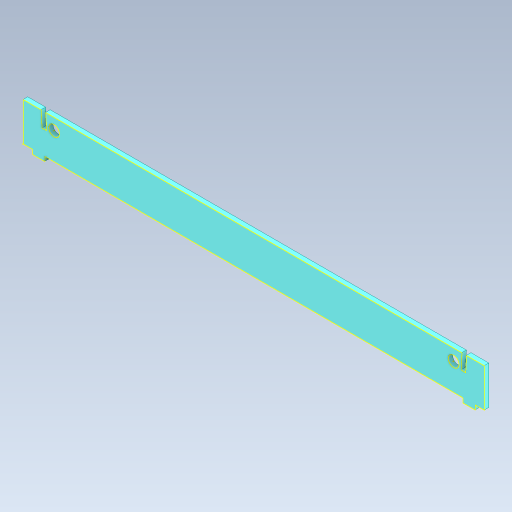
# Autodesk Inventor part: 零件1
Saved by Autodesk Inventor 2023 (Build 270158000, 158)
## iProperties
Created: 2023-04-16
Part Number: 零件1
Material: 一般
Document SubType Name: Modeling
Designer: JOU
Density: 1 g/cm^3
Appearance: 預設
Author: JOU
Autodesk Inventor part; units mm, degrees
ref_plane "YZ Plane" through (0, 0, 0) normal (1, 0, 0) x (0, 1, 0)
ref_plane "XZ Plane" through (0, 0, 0) normal (0, 1, 0) x (-1, 0, 0)
ref_plane "XY Plane" through (0, 0, 0) normal (0, 0, 1) x (1, 0, 0)
sketch "草圖1" plane through (0, 0, 0) normal (0, 0, 1) x (1, 0, 0)
  line L0 (0, 25) -> (300, 25)
  line L1 (300, 25) -> (300, 0)
  line L2 (300, 0) -> (0, 0)
  line L3 (0, 0) -> (0, 25)
  circle A0 centre (20, 17.5) radius 3.5
  circle A1 centre (280, 17.5) radius 3.5
  line L4 (6, 0) -> (14, 0)
  line L5 (14, 0) -> (14, -2.9)
  line L6 (14, -2.9) -> (6, -2.9)
  line L7 (6, -2.9) -> (6, 0)
  line L8 (286, 0) -> (294, 0)
  line L9 (294, 0) -> (294, -2.9)
  line L10 (294, -2.9) -> (286, -2.9)
  line L11 (286, -2.9) -> (286, 0)
  point P0 (6, -1.45)
  point P1 (294, -1.45)
  point P2 (294, 0)
  dimension "d0" = 300
  dimension "d1" = 25
  dimension "d2" = 7.5
  dimension "d3" = 7
  dimension "d4" = 20
  dimension "d5" = 20
  dimension "d6" = 7.5
  dimension "d7" = 7
  dimension "d10" = 6
  dimension "d11" = 6
  dimension "d12" = 8
  dimension "d13" = 2.9
  dimension "d14" = 8
  constraints: 24 end point, 6 parallel, 3 horizontal, 3 perpendicular, 3 point on line, 2 centre point, 2 midpoint, 1 coincident
  measures "d0" distance of L0.start L0.end
  measures "d1" distance of L2.end L0.start
  measures "d2" distance from line of L0 A0.centre
  measures "d3" diameter of A0
  measures "d4" distance from line of L3 A0.centre
  measures "d5" distance from line of A1.centre L1
  measures "d6" distance from line of L0 A1.centre
  measures "d7" diameter of A1
  measures "d10" distance from line of point (6, -1.45) L3
  measures "d11" distance from line of L1 point (294, -1.45)
  measures "d12" distance of L5.end L6.end
  measures "d13" distance of L4.end L5.end
  measures "d14" distance of L9.end L10.end
extrude "擠出1" add sketch "草圖1" along normal blind 3
sketch "草圖2" plane through (0, 0, 3) normal (0, 0, 1) x (1, 0, 0)
  line L0 (11.646, 25) -> (14.592, 25.1544)
  line L1 (14.592, 25.1544) -> (15.1153, 15.1681)
  line L2 (15.1153, 15.1681) -> (12.1694, 15.0137)
  line L3 (12.1694, 15.0137) -> (11.646, 25)
  line L4 (300, 25) -> (0, 25) projected
  line L5 (16.1021, 25) -> (23.0925, 25.3664)
  line L6 (23.0925, 25.3664) -> (24.1149, 5.8596)
  line L7 (24.1149, 5.8596) -> (17.1244, 5.4932)
  line L8 (17.1244, 5.4932) -> (16.1021, 25)
  circle A0 centre (20, 17.5) radius 3.5 projected
  line L9 (15.1153, 15.1681) -> (16.6133, 15.2466)
  line L10 (285.408, 25.1544) -> (288.354, 25)
  line L11 (288.354, 25) -> (287.8306, 15.0137)
  line L12 (287.8306, 15.0137) -> (284.8847, 15.1681)
  line L13 (284.8847, 15.1681) -> (285.408, 25.1544)
  line L14 (276.7474, 22.3122) -> (283.7378, 21.9458)
  line L15 (283.7378, 21.9458) -> (283.1798, 11.2976)
  line L16 (283.1798, 11.2976) -> (276.1893, 11.664)
  line L17 (276.1893, 11.664) -> (276.7474, 22.3122)
  circle A1 centre (280, 17.5) radius 3.5 projected
  line L18 (284.8847, 15.1681) -> (283.3867, 15.2466)
  point P0 (0, 0)
  point P1 (285.3999, 25)
  point P2 (14.6001, 25)
  dimension "d16" = 2.95
  dimension "d18" = 10
  dimension "d19" = 87
  dimension "d20" = 87
  dimension "d21" = 1.5
  dimension "d22" = 87
  dimension "d23" = 87
  dimension "d24" = 2.95
  dimension "d25" = 10
  dimension "d27" = 1.5
  constraints: 36 end point, 8 parallel, 6 perpendicular, 4 point on line, 4 tangent, 1 midpoint
  measures "d16" distance of L0.start L0.end
  measures "d18" distance of L0.end L1.end
  measures "d19" angle of L1 L4
  measures "d20" angle of L6 L4
  measures "d21" distance of L1.end L9.end
  measures "d22" angle of L4 L17
  measures "d23" angle of L4 L13
  measures "d24" distance of L10.start L10.end
  measures "d25" distance of L10.end L11.end
  measures "d27" distance of L12.end L18.end
extrude "擠出2" cut sketch "草圖2" against normal up to surface (3 mm away) contours L4 L1 L2 L3 | L11 L12 L13 L4
sketch "草圖3" plane through (0, 0, 3) normal (0, 0, 1) x (1, 0, 0)
  line L0 (284.8847, 15.1681) -> (285.3999, 25) projected
  line L1 (285.3999, 25) -> (14.6001, 25) projected
  line L2 (14.6001, 25) -> (15.1153, 15.1681) projected
  line L3 (15.1153, 15.1681) -> (12.1694, 15.0137) projected
  line L4 (12.1694, 15.0137) -> (11.646, 25) projected
  line L5 (11.646, 25) -> (0, 25) projected
  line L6 (0, 25) -> (0, 0) projected
  line L7 (0, 0) -> (6, 0) projected
  line L8 (6, 0) -> (6, -2.9) projected
  line L9 (6, -2.9) -> (14, -2.9) projected
  line L10 (14, -2.9) -> (14, 0) projected
  line L11 (14, 0) -> (286, 0) projected
  line L12 (286, 0) -> (286, -2.9) projected
  line L13 (286, -2.9) -> (294, -2.9) projected
  line L14 (294, -2.9) -> (294, 0) projected
  line L15 (294, 0) -> (300, 0) projected
  line L16 (300, 0) -> (300, 25) projected
  line L17 (300, 25) -> (288.354, 25) projected
  line L18 (288.354, 25) -> (287.8306, 15.0137) projected
  line L19 (287.8306, 15.0137) -> (284.8847, 15.1681) projected
  circle A0 centre (280, 17.5) radius 3.5 projected
  circle A1 centre (20, 17.5) radius 3.5 projected
equation "\"d20\" = d19"
equation "\"d22\" = d23"
